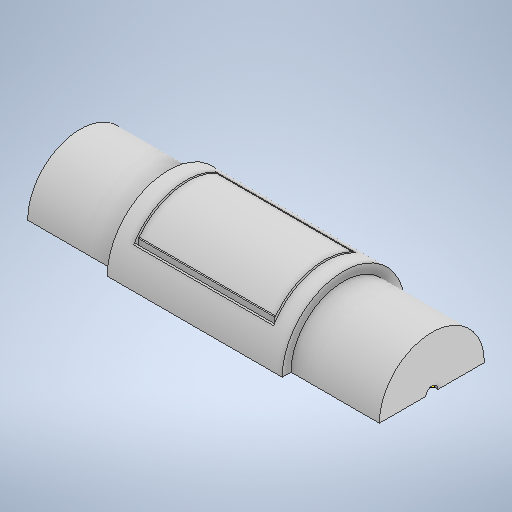
# Autodesk Inventor part: ObereHaelfte
Saved by Autodesk Inventor 2025.2 (Build 292293000, 293)
## iProperties
Created: 2025-04-19
Part Number: ObereHaelfte
Material: Generisch
Document SubType Name: Modeling
Designer: gassl
Density: 1 g/cm^3
Appearance: Vorgabe
Author: gassl
Autodesk Inventor part; units mm, degrees
ref_plane "YZ Plane" through (0, 0, 0) normal (1, 0, 0) x (0, 1, 0)
ref_plane "XZ Plane" through (0, 0, 0) normal (0, 1, 0) x (-1, 0, 0)
ref_plane "XY Plane" through (0, 0, 0) normal (0, 0, 1) x (1, 0, 0)
sketch "Skizze1" plane through (0, 0, 0) normal (1, 0, 0) x (0, 1, 0)
  arc A0 (30, 0) -> (-30, 0) centre (0, 0) ccw
  arc A1 (3.5, 0) -> (-3.5, 0) centre (0, 0) ccw
  line L0 (-30, 0) -> (-3.5, 0)
  line L1 (3.5, 0) -> (30, 0)
  dimension "d0" = 60
  dimension "d1" = 7
  constraints: 4 end point, 4 point on circle, 2 centre point, 2 coincident, 2 horizontal
  measures "d0" diameter of A0
  measures "d1" diameter of A1
extrude "Motorloch R" add sketch "Skizze1" along normal blind 1
sketch "Skizze3" plane through (0, 0, 0) normal (-1, 0, 0) x (0, 0, 1)
  arc A0 (0, -30) -> (0, 30) centre (0, 0) ccw
  line L0 (0, 30) -> (0, -30)
  constraints: 2 end point, 2 point on circle, 1 centre point, 1 coincident, 1 vertical
extrude "Grundkörper R Teil A" add sketch "Skizze3" along normal blind 46
sketch "Skizze4" plane through (-46, 0, 0) normal (-1, 0, 0) x (0, 0, 1)
  arc A0 (0, -35) -> (0, 35) centre (0, 0) ccw
  line L0 (0, 35.8217) -> (0, -35)
  line L1 (0, 3.5) -> (0, 30) projected
  dimension "d8" = 70
  constraints: 2 end point, 2 point on circle, 1 centre point, 1 coincident, 1 collinear, 1 point on line
  measures "d8" diameter of A0
extrude "Grundkörper R Teil B" add sketch "Skizze4" along normal blind 10
sketch "Skizze5" plane through (-56, 0, 0) normal (-1, 0, 0) x (0, 0, 1)
  line L0 (0, -30) -> (0, -35) projected
  line L1 (0, 32.5) -> (0, -35)
  line L2 (0, 35) -> (0, 30) projected
  line L3 (0, 32.5) -> (12.9904, 32.5)
  arc A0 (0, -35) -> (0, 35) centre (0, 0) ccw projected
  line L4 (0, -35) -> (0, -30)
  line L5 (0, -30) -> (0, -3.5) projected
  line L6 (18.0278, -30) -> (30.6125, 16.9669)
  line L7 (18.0278, -30) -> (66.6515, -30) construction
  arc A1 (0, -35) -> (18.0278, -30) centre (0, 0) ccw
  arc A2 (30.6125, 16.9669) -> (12.9904, 32.5) centre (0, 0) ccw
  dimension "d11" = 75
  constraints: 10 end point, 6 point on circle, 2 centre point, 1 coincident, 1 collinear, 1 equal length, 1 horizontal, 1 midpoint, 1 perpendicular, 1 vertical
  measures "d11" angle of L7 L6
extrude "Grundkörper R Teil C" add sketch "Skizze5" along normal blind 15 contours L1 L3 A0 L6 L0
sketch "Skizze6" plane through (-71, 0, 0) normal (-1, 0, 0) x (0, 0, 1)
  line L0 (0, 32.5) -> (0, -35) projected
  line L1 (0, 35) -> (0, -35)
  line L2 (18.0278, -30) -> (30.6125, 16.9669) projected
  line L3 (30.6125, 16.9669) -> (18.0278, -30)
  arc A0 (0, -35) -> (18.0278, -30) centre (0, 0) ccw
  arc A1 (30.6125, 16.9669) -> (0, 35) centre (0, 0) ccw
  constraints: 4 end point, 4 point on circle, 2 centre point, 2 collinear, 1 coincident
extrude "Grundkörper M Teil A" add sketch "Skizze6" along normal blind 50
sketch "Skizze8" plane through (-121, 0, 0) normal (-1, 0, 0) x (0, 0, 1)
  line L0 (0, 32.5) -> (0, -35)
  line L1 (0, -30) -> (0, -3.5) projected
  line L2 (30.6125, 16.9669) -> (18.0278, -30) projected
  line L3 (30.6125, 16.9669) -> (18.0278, -30)
  line L4 (0, 32.5) -> (12.9904, 32.5) projected
  line L5 (0, 32.5) -> (12.9904, 32.5)
  arc A0 (0, -35) -> (18.0278, -30) centre (0, 0) ccw
  arc A1 (30.6125, 16.9669) -> (12.9904, 32.5) centre (0, 0) ccw
  constraints: 6 end point, 4 point on circle, 3 collinear, 2 centre point, 2 point on line, 1 coincident
extrude "Grundkörper L Teil C" add sketch "Skizze8" along normal blind 15
sketch "Skizze9" plane through (-136, 0, 0) normal (-1, 0, 0) x (0, 0, 1)
  arc A0 (0, -35) -> (0, 35) centre (0, 0) ccw
  line L0 (0, 35) -> (0, -35)
  line L1 (0, -30) -> (0, -3.5) projected
  constraints: 2 end point, 2 point on circle, 1 centre point, 1 coincident, 1 collinear
extrude "Grundkörper L Teil B" add sketch "Skizze9" along normal blind 10
sketch "Skizze10" plane through (-146, 0, 0) normal (-1, 0, 0) x (0, 0, 1)
  arc A0 (0, -30) -> (0, 30) centre (0, 0) ccw
  line L0 (0, -30) -> (0, -3.5) projected
  line L1 (0, 30) -> (0, -30)
  constraints: 2 end point, 2 point on circle, 1 centre point, 1 coincident, 1 collinear
extrude "Grundkörper L Teil A" add sketch "Skizze10" along normal blind 46
sketch "Skizze12" plane through (1, 0, 0) normal (1, 0, 0) x (0, 0, -1)
  arc A0 (0, 30) -> (0, -30) centre (0, 0) ccw
  line L0 (0, -30) -> (0, -35) projected
  arc A1 (0, 3.5) -> (0, -3.5) centre (0, 0) ccw
  line L1 (0, -30) -> (0, -3.5)
  line L2 (0, 3.5) -> (0, 30)
  constraints: 4 end point, 4 point on circle, 2 centre point, 2 coincident, 2 collinear
extrude "Grundkörper R Teil D" cut sketch "Skizze12" against normal blind 1
sketch "Skizze13" plane through (-192, 0, 0) normal (-1, 0, 0) x (0, 0, 1)
  line L0 (0, 0) -> (0, -23)
  line L1 (0, 30) -> (0, -30) projected
  line L2 (0, -23) -> (17, -23)
  line L3 (0, 0) -> (0, 23)
  line L4 (0, 23) -> (17, 23)
  line L5 (23, 0) -> (23, -17)
  line L6 (23, 0) -> (23, 17)
  line L7 (23, 17) -> (17, 23)
  line L8 (23, -17) -> (17, -23)
  constraints: 16 end point, 2 point on line, 1 horizontal, 1 perpendicular, 1 vertical
extrude "Motoraushöhlung L" cut sketch "Skizze13" against normal blind 23
sketch "Skizze14" plane through (0, 0, 0) normal (1, 0, 0) x (0, 0, -1)
  line L0 (0, -23) -> (0, 23) projected
  line L1 (0, 0) -> (0, 23)
  line L2 (0, 23) -> (-17, 23) projected
  line L3 (0, 23) -> (-17, 23)
  line L4 (-17, 23) -> (-23, 17)
  line L5 (-23, 17) -> (-23, -17) projected
  line L6 (-23, 17) -> (-23, -17)
  line L7 (-23, -17) -> (-17, -23)
  line L8 (-17, -23) -> (0, -23)
  line L9 (0, -23) -> (0, 0)
  constraints: 14 end point, 4 collinear, 1 parallel, 1 perpendicular, 1 point on line
extrude "Motoraushöhlung R" cut sketch "Skizze14" against normal blind 23
sketch "Skizze16" plane through (-169, 0, 0) normal (-1, 0, 0) x (0, 0, 1)
  line L0 (0, -23) -> (0, -30) projected
  line L1 (0, -23) -> (18, -23)
  line L2 (18, -23) -> (18, 23)
  line L3 (18, 23) -> (0, 23)
  line L4 (0, 23) -> (0, -23)
  point P0 (0, 0)
  dimension "d40" = 18
  dimension "d41" = 46
  constraints: 8 end point, 2 parallel, 1 horizontal, 1 perpendicular
  measures "d40" distance of L3.end L2.end
  measures "d41" distance of L2.end L1.end
extrude "Platienenaushöhlung M" cut sketch "Skizze16" against normal blind 146
sketch "Skizze17" plane through (-136, 16.9669, 30.6125) normal (0, -0.258819, 0.9659258) x (1, 0, 0)
  line L0 (0, 0) -> (0, -48.6237) projected
  line L1 (80, 0) -> (80, -48.6237) projected
  line L2 (0, 0) -> (80, 0)
  line L3 (80, 0) -> (80, -47.5844)
  line L4 (80, -47.5844) -> (0, -47.5844)
  line L5 (0, -47.5844) -> (0, 0)
  point P0 (136, -24.3118)
  constraints: 8 end point, 2 parallel, 1 horizontal, 1 perpendicular, 1 point on line
extrude "LED Klappe Aushöhlung M" cut sketch "Skizze17" against normal blind 13
sketch "Skizze18" plane through (-56, 32.5, 12.9904) normal (0, 1, 0) x (1, 0, 0)
  line L0 (0, 0) -> (-15, 0) projected
  line L1 (10, 12.9904) -> (-90, 12.9904) projected
  line L2 (-80, 6.5456) -> (0, 6.5456) projected
  circle A0 centre (-7.4414, 6.5456) radius 5.1
  line L3 (-7.4996, 6.4952) -> (-7.5578, 6.5456)
  line L4 (-7.4414, 6.5456) -> (-7.4996, 6.4952)
  line L5 (-65, 12.9904) -> (-65, 0) projected
  circle A1 centre (-72.5, 6.4952) radius 5.1
  line L6 (-72.5, 6.4952) -> (-72.5582, 6.5456)
  line L7 (-72.4418, 6.5456) -> (-72.5, 6.4952)
  point P0 (56, 12.9904)
  dimension "d46" = 10.2
  dimension "d47" = 10.2
  constraints: 8 end point, 4 point on line, 2 centre point
  measures "d46" diameter of A0
  measures "d47" diameter of A1
extrude "Kameralöcher" cut sketch "Skizze18" against normal blind 13 contours L2 A1 | L6 L7 L2 A1 | L2 L7 L6 | L2 A0 | L3 L4 L2 A0
sketch "Skizze19" plane through (0, 0, 0) normal (1, 0, 0) x (0, 0, -1)
  arc A0 (0, 30) -> (0, -30) centre (0, 0) ccw
  line L0 (0, -23) -> (0, -30) projected
  arc A1 (0, 3.5) -> (0, -3.5) centre (0, 0) ccw
  line L1 (0, -30) -> (0, -3.5)
  line L2 (0, 3.5) -> (0, 30)
  dimension "d50" = 7
  constraints: 4 end point, 4 point on circle, 2 centre point, 2 coincident, 2 collinear
  measures "d50" diameter of A1
extrude "Grundkörper R Teil E" add sketch "Skizze19" along normal blind 4.5
sketch "Skizze20" plane through (-192, 0, 0) normal (-1, 0, 0) x (0, 0, 1)
  arc A0 (0, -30) -> (0, 30) centre (0, 0) ccw projected
  arc A1 (0, -30) -> (0, 30) centre (0, 0) ccw
  arc A2 (0, -3.5) -> (0, 3.5) centre (0, 0) ccw
  line L0 (0, 35) -> (0, 30) projected
  line L1 (0, 30) -> (0, 3.5)
  line L2 (0, -3.5) -> (0, -30)
  constraints: 4 end point, 4 point on circle, 2 centre point, 2 coincident, 2 collinear
extrude "Grundkörper L Teil E" add sketch "Skizze20" along normal blind 4.5
sketch "Skizze21" plane through (0, 0, 0) normal (-1, 0, 0) x (0, 0, 1)
  arc A0 (0, -3.5) -> (0, 3.5) centre (0, 0) ccw projected
  circle A1 centre (0, 0) radius 11.25
  dimension "d55" = 22.5
  constraints: 1 centre point, 1 coincident
  measures "d55" diameter of A1
extrude "Grundkörper R Teil F" cut sketch "Skizze21" against normal blind 2.5
sketch "Skizze22" plane through (-192, 0, 0) normal (1, 0, 0) x (0, 0, -1)
  circle A0 centre (0, 0) radius 11.25
  dimension "d58" = 22.5
  constraints: 1 centre point, 1 coincident
  measures "d58" diameter of A0
extrude "Grundkörper L Teil F" cut sketch "Skizze22" against normal blind 2.5
sketch "Skizze23" plane through (-56, 0, 0) normal (-1, 0, 0) x (0, 0, 1)
  circle A0 centre (18, -25) radius 1.5
  point P0 (0, 0)
  dimension "d61" = 3
  constraints: 1 centre point
  measures "d61" diameter of A0
extrude "Schanier LED Klappe R" add sketch "Skizze23" along normal blind 10
sketch "Skizze24" plane through (-136, 0, 0) normal (1, 0, 0) x (0, 0, -1)
  circle A0 centre (-18, -25) radius 1.5
  point P0 (0, 0)
  dimension "d64" = 3
  constraints: 1 centre point
  measures "d64" diameter of A0
extrude "Schanier LED Klappe L" add sketch "Skizze24" along normal blind 10
ref_plane "LED Klappe Arbeitsebene" through (-67, -25, 18) normal (-1, 0, 0) x (0, 0, 1)
sketch "Skizze25" plane through (-67, -25, 18) normal (-1, 0, 0) x (0, 0, 1)
  line L0 (-3.25, -3.25) -> (3.25, -3.25)
  line L1 (3.25, -3.25) -> (3.25, 3.25)
  line L2 (3.25, 3.25) -> (-3.25, 3.25)
  line L3 (-3.25, 3.25) -> (-3.25, -3.25)
  circle A0 centre (0, 0) radius 1.5 projected
  line L4 (-3.25, -3.25) -> (3.25, 3.25) construction
  line L5 (3.25, -3.25) -> (-3.25, 3.25) construction
  point P0 (-18, 25)
  dimension "d68" = 6.5
  dimension "d69" = 6.5
  constraints: 12 end point, 2 midpoint, 2 parallel, 1 horizontal, 1 perpendicular
  measures "d68" distance of L2.end L1.end
  measures "d69" distance of L1.end L0.end
extrude "Schanier LED Klappe M" add sketch "Skizze25" along normal blind 58 contours L3 L2 L1 L0 | A0
sketch "Skizze26" plane through (-125, -25, 18) normal (-1, 0, 0) x (0, 0, 1)
  circle A0 centre (0, 0) radius 2
  line L0 (-3.25, 3.25) -> (3.25, 3.25)
  line L1 (3.25, 3.25) -> (3.25, -3.25)
  line L2 (3.25, -3.25) -> (-3.25, -3.25)
  line L3 (-3.25, -3.25) -> (-3.25, 3.25)
  line L4 (-3.25, 3.25) -> (3.25, -3.25) construction
  line L5 (3.25, 3.25) -> (-3.25, -3.25) construction
  point P0 (-18, 25)
  dimension "d72" = 4
  constraints: 12 end point, 2 midpoint, 2 parallel, 1 centre point, 1 horizontal, 1 perpendicular
  measures "d72" diameter of A0
extrude "Schanier LED Klappe M 2" add sketch "Skizze26" along normal blind 10
sketch "Skizze27" plane through (-67, -25, 18) normal (1, 0, 0) x (0, 0, -1)
  circle A0 centre (0, 0) radius 1.5 projected
  circle A1 centre (0, 0) radius 2
  line L0 (3.25, 3.25) -> (-3.25, 3.25)
  line L1 (-3.25, 3.25) -> (-3.25, -3.25)
  line L2 (-3.25, -3.25) -> (3.25, -3.25)
  line L3 (3.25, -3.25) -> (3.25, 3.25)
  line L4 (3.25, 3.25) -> (-3.25, -3.25) construction
  line L5 (-3.25, 3.25) -> (3.25, -3.25) construction
  point P0 (18, 25)
  dimension "d75" = 4
  constraints: 12 end point, 2 midpoint, 2 parallel, 1 centre point, 1 coincident, 1 horizontal, 1 perpendicular
  measures "d75" diameter of A1
extrude "Schanier LED Klappe M 3" add sketch "Skizze27" along normal blind 10 contours L3 L2 L1 L0
sketch "Skizze28" plane through (-135, -28.25, 21.25) normal (0, 0, 1) x (1, 0, 0)
  line L0 (0, 6.5) -> (0, 0.2043) projected
  line L1 (0, 0.2043) -> (78, 0.2043) projected
  line L2 (0, 6.5) -> (78, 6.5)
  line L3 (78, 6.5) -> (78, 0.2043)
  line L4 (78, 0.2043) -> (0, 0.2043)
  line L5 (0, 0.2043) -> (0, 6.5)
  point P0 (135, 28.25)
  constraints: 8 end point, 2 parallel, 1 horizontal, 1 perpendicular
extrude "LED Klappe M Teil A" add sketch "Skizze28" along normal blind 15
sketch "Skizze29" plane through (-135, -21.75, 14.75) normal (0, 1, 0) x (1, 0, 0)
  line L0 (78, -21.5) -> (0, -21.5) projected
  line L1 (78, 0) -> (0, 0) projected
  line L2 (78, -21.5) -> (0, -21.5)
  line L3 (0, -21.5) -> (0, 0)
  line L4 (0, 0) -> (78, 0)
  line L5 (78, 0) -> (78, -21.5)
  point P0 (135, 14.75)
  constraints: 8 end point, 2 parallel, 1 horizontal, 1 perpendicular
extrude "LED Klappe M Teil B" add sketch "Skizze29" along normal blind 37.75
sketch "Skizze30" plane through (-135, -25, 18) normal (-1, 0, 0) x (0, 0, 1)
  arc A0 (-18, -10) -> (-18, 60) centre (-18, 25) ccw projected
  arc A1 (3.2232, -2.8312) -> (13.1347, 40.9885) centre (-18, 25) ccw
  line L0 (18.25, -3.0457) -> (18.25, 41) projected
  line L1 (3.25, -3.0457) -> (3.25, -3.25) projected
  line L2 (18.25, 41) -> (3.25, 41)
  line L3 (3.25, 41) -> (3.25, -3.0457)
  line L4 (3.25, -3.0457) -> (18.25, -3.0457)
  line L5 (18.25, -3.0457) -> (18.25, 41)
  point P0 (13.1288, 41)
  point P1 (3.25, -2.8107)
  constraints: 8 end point, 4 point on circle, 2 parallel, 1 centre point, 1 horizontal, 1 perpendicular
extrude "LED Klappe M Teil C" cut sketch "Skizze30" against normal blind 78.25 contours A0 L2 L0 L4 L3
sketch "Skizze31" plane through (-57, -28.0457, 14.75) normal (0, 0, -1) x (-1, 0, 0)
  line L0 (0, 44.0457) -> (0, 0.235) projected
  line L1 (0, 44.0457) -> (78, 44.0457)
  line L2 (78, 44.0457) -> (78, 5.0457)
  line L3 (78, 5.0457) -> (0, 5.0457)
  line L4 (0, 5.0457) -> (0, 44.0457)
  point P0 (-57, 28.0457)
  point P1 (0, 5.0457)
  dimension "d84" = 78
  dimension "d85" = 39
  constraints: 8 end point, 2 parallel, 1 horizontal, 1 perpendicular
  measures "d84" distance of L2.end L3.end
  measures "d85" distance of L1.end L2.end
extrude "LED Klappe M Aushöhlung" cut sketch "Skizze31" against normal blind 10
sketch "Skizze32" plane through (-135, -28.25, 15.5123) normal (-1, 0, 0) x (0, 0, 1)
  line L0 (5.7377, 0) -> (5.7377, 0.4393) projected
  line L1 (0, 0) -> (5.7377, 0) projected
  line L2 (5.7377, 0.4393) -> (5.7377, 0)
  line L3 (5.7377, 0) -> (5.3729, 0)
  arc A0 (5.3729, 0) -> (5.7377, 0.4393) centre (1.2924, 3.7603) ccw
  point P0 (-15.5123, 28.25)
  constraints: 4 end point, 2 point on circle, 1 centre point, 1 perpendicular, 1 point on line
extrude "LED Klappe M Aushöhlung 2" cut sketch "Skizze32" against normal blind 78
chamfer "LED Klappe M Fase" distance 3 angle 45 1 edges at (-96, -23, 24.75)
sketch "Skizze34" plane through (-46, 35, 0) normal (0, 0, -1) x (-1, 0, 0)
  line L0 (0, -70) -> (0, 0) projected
  line L1 (123, -12) -> (-23, -12) projected
  circle A0 centre (50, -6) radius 4
  point P0 (-46, -35)
  dimension "d95" = 8
  constraints: 1 centre point
  measures "d95" diameter of A0
extrude "Magnethalterung V Aushöhlung" cut sketch "Skizze34" against normal blind 3
chamfer "Magnethalterung V Fase" distance 0.5 angle 45 1 edges at (-92, 29, 0)
